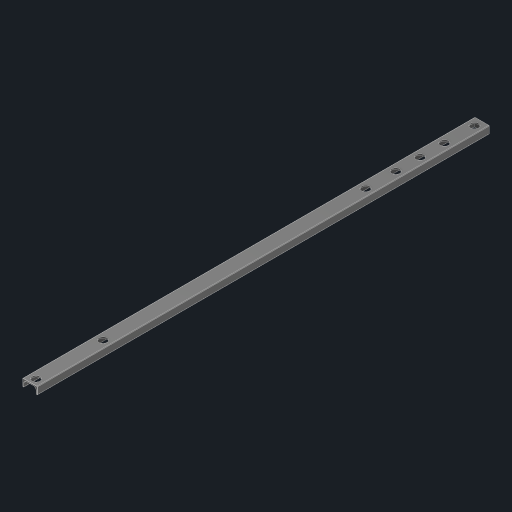
# Autodesk Inventor part: hs_brace_jig
Saved by Autodesk Inventor 2024 (Build 280153000, 153)
## iProperties
Created: 2023-08-26
Part Number: hs_brace_jig
Material: ABS Plastic
Document SubType Name: Modeling
Designer: avere
Density: 1.06 g/cm^3
Appearance: Smooth - White
Author: avere
Autodesk Inventor part; units mm, degrees
ref_plane "YZ Plane" through (0, 0, 0) normal (1, 0, 0) x (0, 1, 0)
ref_plane "XZ Plane" through (0, 0, 0) normal (0, 1, 0) x (-1, 0, 0)
ref_plane "XY Plane" through (0, 0, 0) normal (0, 0, 1) x (1, 0, 0)
sketch "Sketch1" plane through (0, 0, 0) normal (0, 0, 1) x (1, 0, 0)
  line L0 (-2.1082, 3.1877) -> (2.0912, 3.1877)
  line L1 (3.175, 2.1082) -> (3.175, 0.1305)
  line L2 (-3.1877, 0.1305) -> (-3.1877, 2.1082)
  arc A0 (-2.1082, 3.1877) -> (-3.1877, 2.1082) centre (-0.0085, 0.0085) ccw
  line L3 (-2.1082, 3.1877) -> (-3.1877, 2.1082) construction
  line L4 (-2.1082, 3.1877) -> (-0.5816, 3.1877) construction
  arc A1 (3.175, 2.1082) -> (2.0912, 3.1877) centre (-0.0009, 0.0035) ccw
  line L5 (3.8091, 0.0035) -> (3.8091, 3.5595)
  line L6 (3.5551, 3.8135) -> (-3.5569, 3.8135)
  line L7 (-3.8109, 3.5595) -> (-3.8109, 0.0035)
  arc A2 (-3.5569, 3.8135) -> (-3.8109, 3.5595) centre (-3.5569, 3.5595) ccw
  arc A3 (3.8091, 3.5595) -> (3.5551, 3.8135) centre (3.5551, 3.5595) ccw
  line L8 (-3.8109, 0.0035) -> (-3.3147, 0.0035)
  line L9 (3.302, 0.0035) -> (3.8091, 0.0035)
  arc A4 (-3.3147, 0.0035) -> (-3.1877, 0.1305) centre (-3.3147, 0.1305) ccw
  arc A5 (3.175, 0.1305) -> (3.302, 0.0035) centre (3.302, 0.1305) ccw
  point P0 (0, 0)
  point P1 (3.8091, 3.8135)
  point P2 (-3.8109, 3.8135)
  dimension "d0" = 135
  dimension "d1" = 3.81
  dimension "d2" = 3.81
  dimension "d3" = 7.62
  dimension "d4" = 3.81
  dimension "d5" = 0.254
  dimension "d6" = 0.127
  constraints: 20 end point, 12 point on circle, 8 tangent, 6 centre point, 4 horizontal, 4 parallel, 4 point on line, 3 perpendicular, 2 equal radius, 1 equal length
  measures "d0" angle of L3 L4
  measures "d1" radius of A0
  measures "d2" radius of A1
  measures "d3" distance of point (-3.811, 3.813) point (3.809, 3.813)
  measures "d4" distance of point (3.809, 3.813) L5.start
  measures "d5" radius of A2
  measures "d6" radius of A4
extrude "Extrusion1" add sketch "Sketch1" along normal blind 234.95
sketch "Sketch2" plane through (0, 0, 0) normal (0, 0, -1) x (-1, 0, 0)
  line L0 (-3.302, 0.0035) -> (-3.8091, 0.0035) projected
  line L1 (3.5569, 3.8135) -> (-3.5551, 3.8135)
  line L2 (-3.8091, 3.5595) -> (-3.8091, 0.0035)
  line L3 (-3.8091, 0.0035) -> (3.8109, 0.0035)
  line L4 (3.8109, 0.0035) -> (3.8109, 3.5595)
  arc A0 (3.8109, 3.5595) -> (3.5569, 3.8135) centre (3.5569, 3.5595) ccw
  arc A1 (-3.5551, 3.8135) -> (-3.8091, 3.5595) centre (-3.5551, 3.5595) ccw
  point P0 (0, 0)
  dimension "d9" = 0.254
  constraints: 8 end point, 4 point on circle, 4 tangent, 2 centre point, 2 parallel, 1 equal radius, 1 horizontal, 1 perpendicular
  measures "d9" radius of A0
extrude "Extrusion2" add sketch "Sketch2" along normal blind 0.762
sketch "Sketch4" plane through (-0.0085, 3.8135, 0) normal (0, 1, 0) x (1, 0, 0)
  circle A0 centre (0.0085, -3.175) radius 2.0955
  circle A1 centre (0, -231.775) radius 2.0955
  circle A2 centre (0, -196.85) radius 2.0955
  circle A3 centre (0, -59.9694) radius 2.0955
  circle A4 centre (0, -31.5722) radius 2.0955
  circle A5 centre (0, -44.2722) radius 2.0955
  circle A6 centre (0, -18.8722) radius 2.0955
  point P0 (0.0085, 0)
  dimension "d15" = 4.191
  dimension "d16" = 4.191
  dimension "d17" = 4.191
  dimension "d18" = 4.191
  dimension "d19" = 4.191
  dimension "d20" = 4.191
  dimension "d21" = 4.191
  constraints: 7 centre point
  measures "d15" diameter of A0
  measures "d16" diameter of A1
  measures "d17" diameter of A2
  measures "d18" diameter of A3
  measures "d19" diameter of A4
  measures "d20" diameter of A5
  measures "d21" diameter of A6
extrude "Extrusion3" cut sketch "Sketch4" against normal blind 4.191
fillet "Fillet1" radius 0.0762 23 edges at (3.8091, 0.0035, 117.094) (-0.0009, 0.0035, -0.762) (3.7347, 3.7391, -0.762) (-0.0009, 3.8135, -0.762) (-3.7365, 3.7391, -0.762) (-3.8109, 1.7815, -0.762) (3.8091, 1.7815, -0.762) (-3.8109, 0.0035, 117.094) (-0.0063, 0.0035, 0) (3.2122, 0.0407, 234.95) (3.175, 1.1193, 234.95) (3.5556, 0.0035, 234.95) (3.7347, 3.7391, 234.95) (-0.0009, 3.8135, 234.95) (-3.7365, 3.7391, 234.95) (-3.8109, 1.7815, 234.95) (3.8091, 1.7815, 234.95) (2.6878, 2.7029, 234.95) (-0.0085, 3.1877, 234.95) (-2.7026, 2.7026, 234.95) (-3.2249, 0.0407, 234.95) (-3.5628, 0.0035, 234.95) (-3.1877, 1.1193, 234.95)
equation "\"d22\" = d20"
body "Solid1"
